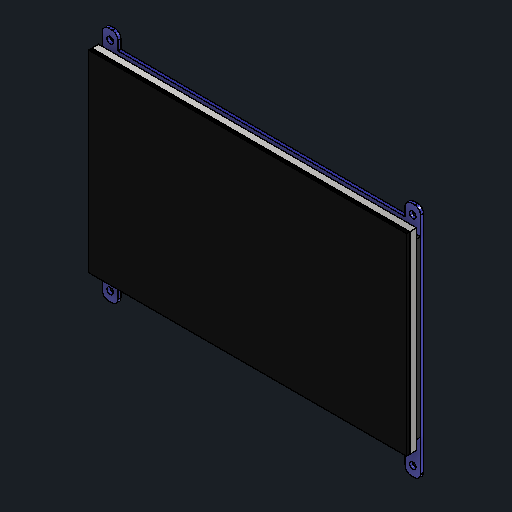
# Autodesk Inventor part: 7in Touch Display
Saved by Autodesk Inventor 2026.2 (Build 302298000, 298)
## iProperties
Created: 2026-01-20
Part Number: 7in Touch Display
Material: Generic
Document SubType Name: Modeling
Designer: JoshuaEah
Density: 1 g/cm^3
Appearance: Default
Author: JoshuaEah
Autodesk Inventor part; units mm, degrees
ref_plane "YZ Plane" through (0, 0, 0) normal (1, 0, 0) x (0, 1, 0)
ref_plane "XZ Plane" through (0, 0, 0) normal (0, 1, 0) x (-1, 0, 0)
ref_plane "XY Plane" through (0, 0, 0) normal (0, 0, 1) x (1, 0, 0)
sketch "Sketch1" plane through (0, 0, 0) normal (0, 0, 1) x (1, 0, 0)
  line L0 (0, 0) -> (164.9, 0)
  line L1 (164.9, 0) -> (164.9, 122.5)
  line L2 (164.9, 122.5) -> (0, 122.5)
  line L3 (0, 122.5) -> (0, 0)
  line L4 (8, 122.5) -> (8, 0)
  line L5 (8, 114.71) -> (156.9, 114.71)
  line L6 (82.45, 122.5) -> (82.45, 0)
  line L7 (0, 61.25) -> (164.9, 61.25)
  line L8 (156.9, 122.5) -> (156.9, 0)
  line L9 (8, 7.79) -> (156.9, 7.79)
  line L10 (4, 117.5) -> (4, 5) construction
  line L11 (4, 117.5) -> (160.9, 117.5) construction
  line L12 (160.9, 117.5) -> (160.9, 5) construction
  line L13 (4, 5) -> (160.9, 5) construction
  circle A0 centre (4, 117.5) radius 1.75
  circle A1 centre (160.9, 117.5) radius 1.75
  circle A2 centre (160.9, 5) radius 1.75
  circle A3 centre (4, 5) radius 1.75
  point P0 (156.9, 0)
  point P1 (156.9, 122.5)
  point P2 (156.9, 115.59)
  dimension "d0" = 164.9
  dimension "d1" = 122.5
  dimension "d18" = 106.92
  dimension "d21" = 156.9
  dimension "d22" = 112.5
  dimension "d23" = 3.5
  dimension "d24" = 148.9
  constraints: 28 end point, 8 symmetric about line, 4 centre point, 4 coincident, 4 midpoint, 4 point on line, 3 equal radius, 3 parallel, 2 perpendicular, 1 horizontal, 1 vertical
  measures "d0" distance of L2.end L1.end
  measures "d1" distance of L1.end L0.end
  measures "d18" diameter of L5 L7
  measures "d21" diameter of L10 L6
  measures "d22" diameter of L11 L7
  measures "d23" diameter of A0
  measures "d24" diameter of L4 L6
extrude "Extrusion1" add sketch "Sketch1" against normal blind 1.56 contours L3 L7 L4 L0 | L3 L2 L4 L7 | L4 L7 L6 L9 | L4 L5 L6 L7 | L8 L7 L1 L0 | L6 L7 L8 L9 | L6 L5 L8 L7 | L8 L2 L1 L7 | A0 | A1 | A2 | A3
fillet "Fillet1" radius 3 8 edges at (0, 122.5, -0.78) (8, 122.5, -0.78) (156.9, 122.5, -0.78) (164.9, 122.5, -0.78) (0, 0, -0.78) (8, 0, -0.78) (156.9, 0, -0.78) (164.9, 0, -0.78)
hole "Hole1" at (4, 117.5, 0) at (160.9, 117.5, 0) at (160.9, 5, 0) at (4, 5, 0) direction (0, 0, -1) diameter 3.4 end through all clearance for "Flat Head Machine Screw" size "M3" standard "Ansi Metric M Profile"
sketch "Sketch3" plane through (0, 0, 0) normal (0, 0, 1) x (1, 0, 0)
  line L0 (0, 114.71) -> (164.9, 114.71)
  line L1 (164.9, 114.71) -> (164.9, 14.79)
  line L2 (164.9, 14.79) -> (0, 14.79)
  line L3 (0, 14.79) -> (0, 114.71)
  line L4 (0, 119.5) -> (0, 3) construction
  line L5 (164.9, 3) -> (164.9, 119.5) projected
  line L6 (156.9, 114.71) -> (8, 114.71) construction
  line L7 (15, 114.71) -> (15, 14.79)
  line L8 (82.45, 114.71) -> (82.45, 14.79)
  line L9 (149.9, 114.71) -> (149.9, 14.79)
  line L10 (0, 109.71) -> (164.9, 109.71)
  line L11 (164.9, 61.25) -> (0, 61.25)
  line L12 (0, 19.71) -> (164.9, 19.71)
  line L13 (8, 7.79) -> (156.9, 7.79) projected
  point P0 (156.9, 115.59)
  point P1 (8, 114.71)
  point P2 (149.9, 114.71)
  point P3 (149.9, 14.79)
  point P4 (15, 109.71)
  point P5 (0, 109.71)
  point P6 (0, 19.71)
  point P7 (15, 19.71)
  point P8 (149.9, 109.71)
  point P9 (149.9, 19.71)
  point P10 (164.9, 19.71)
  dimension "d38" = 15
  dimension "d43" = 5
  dimension "d44" = 90
  dimension "d45" = 7
  constraints: 20 end point, 8 point on line, 4 perpendicular, 3 midpoint, 2 parallel, 2 symmetric about line, 1 horizontal, 3 other
  measures "d38" distance between parallel lines of L7 L3
  measures "d43" distance between parallel lines of L0 L10
  measures "d44" distance between parallel lines of L10 L12
  measures "d45" distance between parallel lines of L2 L13
extrude "Extrusion2" add sketch "Sketch3" along normal blind 2.04 separate body contours L10 L7 L11 L3 | L11 L7 L12 L3 | L10 L1 L11 L9 | L11 L1 L12 L9
extrude "Extrusion3" add sketch "Sketch3" along normal blind 3.45 from surface at 2.04 separate body
extrude "Extrusion4" add sketch "Sketch3" along normal blind 1.75 from surface at 5.49 separate body
